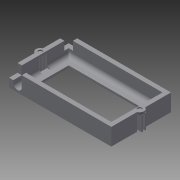
# Autodesk Inventor part: battery clip v1
Saved by Autodesk Inventor 2014 SP1 (Build 180222100, 222)
## iProperties
Created: 2017-06-21
Part Number: battery clip v1
Material: Generic
Document SubType Name: Modeling
Designer: kteo17
Density: 1 g/cm^3
Appearance: Default
Author: kteo17
Autodesk Inventor part; units mm, degrees
ref_plane "YZ Plane" through (0, 0, 0) normal (1, 0, 0) x (0, 1, 0)
ref_plane "XZ Plane" through (0, 0, 0) normal (0, 1, 0) x (-1, 0, 0)
ref_plane "XY Plane" through (0, 0, 0) normal (0, 0, 1) x (1, 0, 0)
sketch "Sketch1" plane through (0, 0, 0) normal (0, 0, 1) x (1, 0, 0)
  line L0 (0, 0) -> (0, 76.2)
  line L1 (44.45, 76.2) -> (44.45, 0)
  arc A0 (25.2062, 76.2) -> (19.2438, 76.2) centre (22.225, 75.1078) ccw
  arc A1 (19.2438, 0) -> (25.2062, 0) centre (22.225, 1.0922) ccw
  line L2 (44.45, 0) -> (25.2062, 0)
  line L3 (19.2438, 0) -> (0, 0)
  line L4 (0, 76.2) -> (19.2438, 76.2)
  line L5 (25.2062, 76.2) -> (44.45, 76.2)
  dimension "d1" = 76.2
  dimension "d7" = 6.35
  dimension "d8" = 6.35
  dimension "d9" = 74.0156
  dimension "d10" = 44.45
  constraints: 12 end point, 5 parallel, 4 point on circle, 2 centre point, 2 perpendicular, 1 vertical
  measures "d1" distance of L1.start L1.end
  measures "d7" diameter of A0
  measures "d8" diameter of A1
  measures "d9" distance of A1.centre A0.centre
  measures "d10" distance between parallel lines of L1 L0
extrude "Extrusion1" add sketch "Sketch1" along normal blind 12.7
sketch "Sketch2" plane through (0, 0, 12.7) normal (0, 0, 1) x (1, 0, 0)
  arc A0 (19.2438, 0) -> (25.2062, 0) centre (22.225, 1.0922) ccw projected
  arc A1 (25.2062, 76.2) -> (19.2438, 76.2) centre (22.225, 75.1078) ccw projected
  line L0 (41.275, 73.025) -> (41.275, 3.175)
  line L1 (3.175, 3.175) -> (3.175, 73.025)
  line L2 (41.275, 3.175) -> (25.2062, 3.175)
  line L3 (19.2438, 3.175) -> (3.175, 3.175)
  line L4 (3.175, 73.025) -> (19.2438, 73.025)
  line L5 (25.2062, 73.025) -> (41.275, 73.025)
  line L6 (19.2438, 76.2) -> (0, 76.2) projected
  line L7 (19.2438, 73.025) -> (25.2062, 73.025)
  line L8 (19.2438, 3.175) -> (25.2062, 3.175)
  point P0 (25.2062, 0)
  constraints: 16 end point, 6 parallel, 2 horizontal, 2 perpendicular, 1 collinear, 1 point on circle
extrude "Extrusion2" cut sketch "Sketch2" against normal blind 11.1125
sketch "Sketch3" plane through (0, 0, 1.5875) normal (0, 0, 1) x (1, 0, 0)
  line L0 (9.525, 66.675) -> (34.925, 66.675)
  line L1 (34.925, 66.675) -> (34.925, 9.525)
  line L2 (34.925, 9.525) -> (9.525, 9.525)
  line L3 (9.525, 9.525) -> (9.525, 66.675)
  point P0 (0, 0)
  constraints: 8 end point, 2 parallel, 1 horizontal, 1 perpendicular
extrude "Extrusion3" cut sketch "Sketch3" against normal blind 1.5875
sketch "Sketch4" plane through (0, 0, 0) normal (0, 0, -1) x (-1, 0, 0)
  arc A0 (-19.2438, 76.2) -> (-25.2062, 76.2) centre (-22.225, 75.1078) ccw projected
  arc A1 (-25.2062, 0) -> (-19.2438, 0) centre (-22.225, 1.0922) ccw projected
  circle A2 centre (-22.225, 75.1078) radius 1.5875
  circle A3 centre (-22.225, 1.0922) radius 1.5875
  dimension "d19" = 3.175
  dimension "d20" = 3.175
  constraints: 2 centre point, 2 coincident
  measures "d19" diameter of A2
  measures "d20" diameter of A3
extrude "Extrusion4" cut sketch "Sketch4" against normal blind 0.7937
sketch "Sketch5" plane through (0, 0, 0) normal (0, 0, -1) x (-1, 0, 0)
  arc A0 (-19.2438, 76.2) -> (-25.2062, 76.2) centre (-22.225, 75.1078) ccw projected
  arc A1 (-25.2062, 0) -> (-19.2438, 0) centre (-22.225, 1.0922) ccw projected
  line L0 (-19.2438, 0) -> (0, 0) projected
  line L1 (-25.2062, 0) -> (-25.2062, 3.175)
  line L2 (-25.2062, 3.175) -> (-19.2438, 3.175)
  line L3 (-19.2438, 3.175) -> (-19.2438, 0)
  line L4 (-19.2438, 76.2) -> (-19.2438, 73.025)
  line L5 (-19.2438, 73.025) -> (-25.2062, 73.025)
  line L6 (-25.2062, 73.025) -> (-25.2062, 76.2)
  constraints: 12 end point, 3 equal length, 3 perpendicular, 1 point on circle
extrude "Extrusion5" cut sketch "Sketch5" against normal blind 11.1125
sketch "Sketch6" plane through (0, 0, 12.7) normal (0, 0, 1) x (1, 0, 0)
  arc A0 (19.2438, 0) -> (25.2062, 0) centre (22.225, 1.0922) ccw projected
  arc A1 (25.2062, 76.2) -> (19.2438, 76.2) centre (22.225, 75.1078) ccw projected
  circle A2 centre (22.225, 75.1078) radius 1.5875
  circle A3 centre (22.225, 1.0922) radius 1.5875
  dimension "d25" = 3.175
  dimension "d26" = 3.175
  constraints: 2 centre point, 2 coincident
  measures "d25" diameter of A2
  measures "d26" diameter of A3
extrude "Extrusion6" cut sketch "Sketch6" against normal blind 0.7937
sketch "Sketch7" plane through (0, 0, 11.1125) normal (0, 0, -1) x (-1, 0, 0)
  line L0 (-23.8125, 0) -> (-23.8125, -2.0828)
  line L1 (-20.6375, -2.0828) -> (-20.6375, 0)
  line L2 (-21.4375, 0) -> (-21.4375, 2.775)
  line L3 (-20.6375, 2.775) -> (-20.6375, 0)
  line L4 (-23.0125, 0) -> (-23.0125, 2.775)
  line L5 (-23.8125, 2.775) -> (-23.8125, 0)
  line L6 (-20.6375, 2.775) -> (-21.4375, 2.775)
  line L7 (-23.0125, 2.775) -> (-23.8125, 2.775)
  line L8 (-21.4375, 0) -> (-21.4375, -2.0828)
  line L9 (-23.0125, -2.0828) -> (-23.0125, 0)
  line L10 (-23.8125, -2.0828) -> (-23.0125, -2.0828)
  line L11 (-21.4375, -2.0828) -> (-20.6375, -2.0828)
  line L12 (-23.8125, 76.2) -> (-23.8125, 78.2828)
  line L13 (-20.6375, 78.2828) -> (-20.6375, 76.2)
  line L14 (-21.4375, 76.2) -> (-21.4375, 73.425)
  line L15 (-20.6375, 73.425) -> (-20.6375, 76.2)
  line L16 (-23.0125, 76.2) -> (-23.0125, 73.425)
  line L17 (-23.8125, 73.425) -> (-23.8125, 76.2)
  line L18 (-20.6375, 73.425) -> (-21.4375, 73.425)
  line L19 (-23.0125, 73.425) -> (-23.8125, 73.425)
  line L20 (-21.4375, 76.2) -> (-21.4375, 78.2828)
  line L21 (-23.0125, 78.2828) -> (-23.0125, 76.2)
  line L22 (-23.8125, 78.2828) -> (-23.0125, 78.2828)
  line L23 (-21.4375, 78.2828) -> (-20.6375, 78.2828)
  point P0 (-25.2062, 0)
  point P1 (-19.2438, 0)
  point P2 (-19.2438, 3.175)
  point P3 (-25.2062, 3.175)
  point P4 (-22.225, 1.0922)
  point P5 (0, 0)
  constraints: 48 end point, 4 parallel, 3 perpendicular
extrude "Extrusion7" add sketch "Sketch7" along normal blind 11.1125
sketch "Sketch8" plane through (0, 0, 12.7) normal (0, 0, 1) x (1, 0, 0)
  line L0 (3.175, 3.175) -> (3.175, 73.025) projected
  line L1 (0, 76.2) -> (0, 0) projected
  line L2 (0, 73.025) -> (3.175, 73.025)
  line L3 (3.175, 73.025) -> (3.175, 66.675)
  line L4 (3.175, 66.675) -> (0, 66.675)
  line L5 (0, 66.675) -> (0, 73.025)
  constraints: 8 end point, 2 parallel, 2 point on line, 1 horizontal, 1 perpendicular
extrude "Extrusion8" cut sketch "Sketch8" against normal blind 11.1125
sketch "Sketch9" plane through (0, 0, 12.7) normal (0, 0, 1) x (1, 0, 0)
  line L0 (0, 73.025) -> (41.275, 73.025) projected
  line L1 (41.275, 73.025) -> (41.275, 3.175) projected
  line L2 (44.45, 0) -> (44.45, 76.2) projected
  line L3 (44.45, 76.2) -> (25.2062, 76.2) projected
  line L4 (0, 76.2) -> (6.35, 76.2)
  line L5 (6.35, 76.2) -> (6.35, 73.025)
  line L6 (6.35, 73.025) -> (0, 73.025)
  line L7 (0, 73.025) -> (0, 76.2)
  line L8 (38.1, 76.2) -> (44.45, 76.2)
  line L9 (44.45, 76.2) -> (44.45, 69.85)
  line L10 (44.45, 69.85) -> (41.275, 69.85)
  line L11 (38.1, 76.2) -> (38.1, 73.025)
  line L12 (41.275, 73.025) -> (41.275, 69.85)
  line L13 (41.275, 73.025) -> (38.1, 73.025)
  constraints: 20 end point, 5 point on line, 3 collinear, 3 perpendicular, 2 parallel, 1 horizontal
extrude "Extrusion9" cut sketch "Sketch9" against normal blind 6.35
fillet "Fillet4" radius 3.175 7 edges at (9.6219, 73.025, 1.5875) (33.2406, 73.025, 1.5875) (41.275, 38.1, 1.5875) (3.175, 34.925, 1.5875) (11.2094, 3.175, 1.5875) (33.2406, 3.175, 1.5875) (1.5875, 66.675, 1.5875)
body "Solid1"
